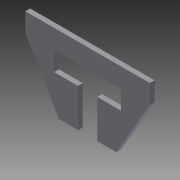
# Autodesk Inventor part: HW 2 Part 1
Saved by Autodesk Inventor 2015 SP1 (Build 190203100, 203)
## iProperties
Created: 2016-01-20
Part Number: HW 2 Part 1
Material: Generic
Document SubType Name: Modeling
Designer: melissa.roth
Density: 1 g/cm^3
Appearance: Default
Author: melissa.roth
Autodesk Inventor part; units mm, degrees
ref_plane "YZ Plane" through (0, 0, 0) normal (1, 0, 0) x (0, 1, 0)
ref_plane "XZ Plane" through (0, 0, 0) normal (0, 1, 0) x (-1, 0, 0)
ref_plane "XY Plane" through (0, 0, 0) normal (0, 0, 1) x (1, 0, 0)
sketch "Sketch1" plane through (0, 0, 0) normal (0, 0, 1) x (1, 0, 0)
  line L0 (0, 0) -> (0, 25.4)
  line L1 (0, 25.4) -> (165.1, 25.4)
  line L2 (165.1, 25.4) -> (165.1, 0)
  line L3 (165.1, 0) -> (120.65, -76.2)
  line L4 (120.65, -76.2) -> (95.25, -76.2)
  line L5 (95.25, -76.2) -> (95.25, -25.4)
  line L6 (95.25, -25.4) -> (127, -25.4)
  line L7 (127, -25.4) -> (127, 0)
  line L8 (127, 0) -> (38.1, 0)
  line L9 (38.1, 0) -> (38.1, -25.4)
  line L10 (38.1, -25.4) -> (69.85, -25.4)
  line L11 (69.85, -25.4) -> (69.85, -76.2)
  line L12 (69.85, -76.2) -> (44.45, -76.2)
  line L13 (44.45, -76.2) -> (0, 0)
  dimension "d0" = 165.1
  dimension "d1" = 120.65
  dimension "d2" = 44.45
  dimension "d3" = 69.85
  dimension "d5" = 25.4
  dimension "d6" = 25.4
  dimension "d7" = 101.6
  dimension "d8" = 101.6
  dimension "d9" = 88.9
  dimension "d11" = 25.4
  dimension "d12" = 38.1
  dimension "d13" = 38.1
  dimension "d14" = 25.4
  dimension "d15" = 25.4
  dimension "d16" = 90
  constraints: 28 end point, 6 perpendicular, 1 parallel
  measures "d0" distance of L0.end L1.end
  measures "d1" horizontal distance of L3.end L0.start
  measures "d2" horizontal distance of L12.end L0.start
  measures "d3" horizontal distance of L11.end L0.start
  measures "d5" distance of L7.end L6.end
  measures "d6" distance between parallel lines of L1 L8
  measures "d7" vertical distance of L12.end L0.end
  measures "d8" vertical distance of L3.end L1.end
  measures "d9" distance of L7.end L8.end
  measures "d11" distance between parallel lines of L5 L11
  measures "d12" horizontal distance of L0.end L8.end
  measures "d13" horizontal distance of L1.end L7.end
  measures "d14" distance of L0.end L0.start
  measures "d15" distance of L1.end L2.end
  measures "d16" angle of L1 L0
extrude "Extrusion1" add sketch "Sketch1" along normal blind 6.35
body "Solid1"
